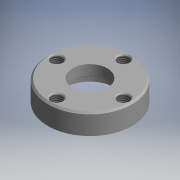
# Autodesk Inventor part: 1559396 EAGF-V2-KF-100---(R)
Saved by Autodesk Inventor 2017.3 (Build 213256000, 256)
## iProperties
Part Number: 1559396 EAGF-V2-KF-100---(R)
Material: Generic
Catalog Web Link: www.cadenas.de
Description: EAGF-V2-KF-(R)-Ring
Vendor: FESTO
Document SubType Name: Modeling
Designer: partserver
Manufacturer: FESTO
Mass: 61.2064 g
Surface Area: 162.591 cm^2
Volume: 61.2064 cm^3
Density: 1 g/cm^3
Appearance: PSOLRGB-192-192-192
Category: PARTsolutions
Company: FESTO
Title: 1559396 EAGF-V2-KF-100---(R)
Author: Cadenas PARTsolutions
Comments: Ring
PSOL_IDENT_0: {$CADENAS_DATA\23d-libs\festo\parts\e\eagf\parts\eagf_ring.prj},204 {VTYP=3D},{NB=1559396 EAGF-V2-KF
PSOL_IDENT_1: -100---(R)},{LINA=1559396 EAGF-V2-KF-100---(R)},{NN=EAGF-V2-KF-(R)},{DATE=20.07.2020 13:53:58},{GEOM
PSOL_IDENT_2: DATE=17.05.2016 08:00:00},{VERSION=},{LINEID=60},{WBVAR=},{WBNUMERIC=}  {NB=1559396 EAGF-V2-KF-100--
PSOL_IDENT_3: -(R)},{LINA=1559396 EAGF-V2-KF-100---(R)},{KT=DUMMY},{TNR=1559396},{TYP=EAGF-V2-KF-100},{KDM=100},{D
PSOL_IDENT_4: 1=78.000},{D2=62.000},{D3=46.000},{D4=32.000},{D5=12.000},{D6=0.000},{D7=0.000},{H=19.000},{T1=9.050
PSOL_IDENT_5: },{ANZ=4.000},{W=90.000}
NB: 1559396 EAGF-V2-KF-100---(R)
NN: EAGF-V2-KF-(R)
NT: Ring
NBSYN: $TNR. $TYP.---(R)
LINA: 1559396 EAGF-V2-KF-100---(R)
CATALOG: Festo
TNR: 1559396
TYP: EAGF-V2-KF-100
KDM: 100
D1: 78
D2: 62
D3: 46
D4: 32
D5: 12
D6: 0
D7: 0
H: 19
T1: 9.05
ANZ: 4
W: 90
SUPPLIER: FESTO
ARTICLENO: 1559396 EAGF-V2-KF-100---(R)
BOMINFO: 1559396 EAGF-V2-KF-100---(R)
CREATOR: CADENAS GmbH
Autodesk Inventor part; units mm, degrees
sketch "Sketch_1" plane through (0, 0, 0) normal (1, 0, 0) x (0, 1, 0)
  line L0 (0, -19) -> (0, 0)
  line L1 (23, 0) -> (23, -8.65)
  arc A0 (22.6, -9.05) -> (23, -8.65) centre (22.6, -8.65) ccw
  line L2 (22.6, -9.05) -> (16.6, -9.05)
  line L3 (16.6, -9.05) -> (16, -9.65)
  line L4 (16, -9.65) -> (16, -19)
  line L5 (16, -19) -> (37.4, -19)
  line L6 (37.4, -19) -> (39, -17.4)
  line L7 (39, -17.4) -> (39, 0)
  line L8 (39, 0) -> (23, 0)
  constraints: 18 end point, 2 point on circle, 1 centre point
revolve "Revolution1" add sketch "Sketch_1" angle 360 about axis through (0, 0, -19) along (0, 0, -1)
sketch "Sketch_2" plane through (0, 0, 0) normal (1, 0, 0) x (0, 1, 0)
  line L0 (31, -19) -> (31, 0)
  line L1 (31, 0) -> (37, 0)
  line L2 (37, 0) -> (36.053, -0.947)
  line L3 (36.053, -0.947) -> (36.053, -18.053)
  line L4 (36.053, -18.053) -> (37, -19)
  line L5 (37, -19) -> (31, -19)
  line L6 (31, -19) -> (31, 0)
  constraints: 14 end point
revolve "Revolution2" cut sketch "Sketch_2" angle 360 about axis through (0, 31, -19) along (0, 0, -1)
thread "Thread1" size "M12x1.75" class "6H" standard "ISO Metric profile" full length
pattern_linear "Rectangular Pattern1" count 2 spacing 43.8406 along (-0.7071, -0.7071, 0) count 2 spacing 43.8406 along (0.7071, -0.7071, 0) of "Revolution2"
ref_plane "ANBAU_XY" through (0, 0, 0) normal (0, 0, 1) x (1, 0, 0)
ref_plane "ANBAU_YZ" through (0, 0, 0) normal (1, 0, 0) x (0, 1, 0)
ref_plane "ANBAU_ZX" through (0, 0, 0) normal (0, 1, 0) x (0, 0, 1)
ref_plane "EP_IP_XY" through (0, 0, -9.05) normal (0, 0, -1) x (1, 0, 0)
ref_plane "EP_IP_YZ" through (0, 0, -9.05) normal (1, 0, 0) x (0, -1, 0)
ref_plane "EP_IP_ZX" through (0, 0, -9.05) normal (0, -1, 0) x (0, 0, -1)
body "Solid1"
